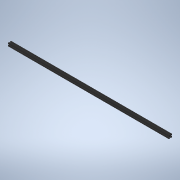
# Autodesk Inventor part: 25.01.1300(00-00-0)(0)
Saved by Autodesk Inventor 2021 (Build 250183000, 183)
## iProperties
Created: 2025-04-03
Part Number: 25.01.1300(00-00-0)(0)
Material: Generic
Catalog Web Link: www.cadenas.de
Description: Aluminium Profile mk 2025.01-Aluminium Construction Profiles Series 25
Vendor: MASCHINENBAUKITZ
Document SubType Name: Modeling
Designer: psAdmin
Manufacturer: MASCHINENBAUKITZ
Mass: 975 g
Surface Area: 3416.74 cm^2
Volume: 363.268 cm^3
Density: 1 g/cm^3
Appearance: PSOLRGB-175-175-175
Category: PARTsolutions
Company: MASCHINENBAUKITZ
Title: 25.01.1300(00-00-0)
Author: Cadenas PARTsolutions
Comments: Aluminium Construction Profiles Series 25
L: 1300
PSOL_IDENT_0: {$CADENAS_DATA/23d-libs/maschinenbau_kitz/1_profiltechnik/1_profile/1_serie25/mk_2025_01.prj},247 {V
PSOL_IDENT_1: TYP=3D},{NB=25.01.1300(00-00-0)(0)},{LINA=25.01.1300(00-00-0)},{NN=Aluminium Profile mk 2025.01},{DA
PSOL_IDENT_2: TE=17.07.2024 10:27:50},{GEOMDATE=19.01.2024 09:39:34},{VERSION=},{LINEID=10},{WBVAR=L,MOD,ALPHA,BET
PSOL_IDENT_3: A,POS,DARST},{WBNUMERIC=L,ALPHA,BETA,DARST}  {NB=25.01.1300(00-00-0)(0)},{LINA=25.01.1300(00-00-0)},
PSOL_IDENT_4: {KT=DUMMY},{ARTIKELNR=25.01.},{L=1300},{MOD=-},{ALPHA=0},{BETA=0},{POS=-},{POSALG='-','none','../../
PSOL_IDENT_5: pics/pos_none.png'},{DARST=0},{GW=0.75},{BZ1=Profil mk 2025.01},{MTR=AlMgSi 0,5 F25},{OBRFL=eloxiert
PSOL_IDENT_6: E6/EV1},{ABM=25 x 25 mm},{FRB=Alu natur},{LGL=5100},{A=279.13},{IX=1.73},{IY=1.73},{WX=1.38},{WY=1.
PSOL_IDENT_7: 38},{O=},{GWCALC=0.975},{ALPHAALG=[0:0]},{BETAALG=[0:0]},{LINAALG=25.01.1300(00-00-0)}
NB: 25.01.1300(00-00-0)(0)
NN: Aluminium Profile mk 2025.01
NT: Aluminium Construction Profiles Series 25
NBSYN: $LINAALG.($DARST.)
LINA: 25.01.1300(00-00-0)
CATALOG: Maschinenbau Kitz
ARTIKELNR: 25.01.
MOD: none
ALPHA: 0
BETA: 0
POS: none
DARST: High
GW: 0.75
BZ1: Profile mk 2025.01
MTR: AlMgSi 0,5 F25
OBRFL: anodized E6/EV1
ABM: 25 x 25 mm
FRB: Alu natural
LGL: 5100
A: 279.13
IX: 1.73
IY: 1.73
WX: 1.38
WY: 1.38
SUPPLIER: MASCHINENBAUKITZ
ARTICLENO: 25.01.1300(00-00-0)(0)
BOMINFO: 25.01.1300(00-00-0)
CREATOR: CADENAS GmbH
Autodesk Inventor part; units mm, degrees
ref_plane "YZ Plane" through (0, 0, 0) normal (1, 0, 0) x (0, 1, 0)
ref_plane "XZ Plane" through (0, 0, 0) normal (0, 1, 0) x (-1, 0, 0)
ref_plane "XY Plane" through (0, 0, 0) normal (0, 0, 1) x (1, 0, 0)
sketch "Skizze_1" plane through (0, 0, 0) normal (1, 0, 0) x (0, 1, 0)
  line L0 (0, 0) -> (0, -9.475)
  line L1 (0, -9.475) -> (2, -9.475)
  line L2 (2, -9.475) -> (2, -7.25)
  line L3 (2, -7.25) -> (5.5, -7.25)
  line L4 (5.5, -7.25) -> (6.5, -8.25)
  line L5 (6.5, -8.25) -> (6.5, -16.75)
  line L6 (6.5, -16.75) -> (5.5, -17.75)
  line L7 (5.5, -17.75) -> (2, -17.75)
  line L8 (2, -17.75) -> (2, -15.525)
  line L9 (2, -15.525) -> (0, -15.525)
  line L10 (0, -15.525) -> (0, -25)
  line L11 (0, -25) -> (9.475, -25)
  line L12 (9.475, -25) -> (9.475, -23)
  line L13 (9.475, -23) -> (7.25, -23)
  line L14 (7.25, -23) -> (7.25, -19.5)
  line L15 (7.25, -19.5) -> (8.25, -18.5)
  line L16 (8.25, -18.5) -> (16.75, -18.5)
  line L17 (16.75, -18.5) -> (17.75, -19.5)
  line L18 (17.75, -19.5) -> (17.75, -23)
  line L19 (17.75, -23) -> (15.525, -23)
  line L20 (15.525, -23) -> (15.525, -25)
  line L21 (15.525, -25) -> (25, -25)
  line L22 (25, -25) -> (25, -15.525)
  line L23 (25, -15.525) -> (23, -15.525)
  line L24 (23, -15.525) -> (23, -17.75)
  line L25 (23, -17.75) -> (19.5, -17.75)
  line L26 (19.5, -17.75) -> (18.5, -16.75)
  line L27 (18.5, -16.75) -> (18.5, -8.25)
  line L28 (18.5, -8.25) -> (19.5, -7.25)
  line L29 (19.5, -7.25) -> (23, -7.25)
  line L30 (23, -7.25) -> (23, -9.475)
  line L31 (23, -9.475) -> (25, -9.475)
  line L32 (25, -9.475) -> (25, 0)
  line L33 (25, 0) -> (15.525, 0)
  line L34 (15.525, 0) -> (15.525, -2)
  line L35 (15.525, -2) -> (17.75, -2)
  line L36 (17.75, -2) -> (17.75, -5.5)
  line L37 (17.75, -5.5) -> (16.75, -6.5)
  line L38 (16.75, -6.5) -> (8.25, -6.5)
  line L39 (8.25, -6.5) -> (7.25, -5.5)
  line L40 (7.25, -5.5) -> (7.25, -2)
  line L41 (7.25, -2) -> (9.475, -2)
  line L42 (9.475, -2) -> (9.475, 0)
  line L43 (9.475, 0) -> (0, 0)
  circle A0 centre (3.75, -21.25) radius 2.1
  circle A1 centre (21.25, -21.25) radius 2.1
  circle A2 centre (12.5, -12.5) radius 4.25
  circle A3 centre (3.75, -3.75) radius 2.1
  circle A4 centre (21.25, -3.75) radius 2.1
  constraints: 88 end point, 5 centre point
extrude "Extrusion1" add sketch "Skizze_1" along normal blind 1300
equation "\"d0\" = L"
equation "\"L\" = 1300"
body "Solid1"
